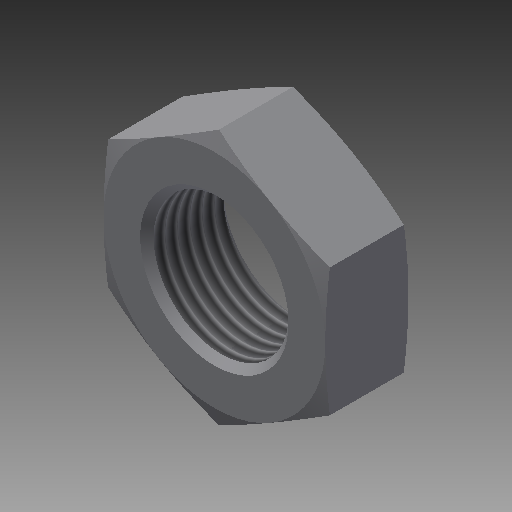
# Autodesk Inventor part: D-3556
Saved by Autodesk Inventor 2019 (Build 230136000, 136)
## iProperties
Category: PARTsolutions
Company: BIMBA
Created: 2019-01-13
Part Number: D-3556
Material: Generic
Catalog Web Link: www.cadenas.de
Description: Mounting Nut for Original Line Cylinders-
Vendor: BIMBA
Document SubType Name: Modeling
Designer: psadmin
Manufacturer: BIMBA
Mass: 4.89558 g
Surface Area: 24.7389 cm^2
Volume: 4.89558 cm^3
Density: 1 g/cm^3
Appearance: PSOLRGB-191-191-191
PSOL_IDENT_0: {$CADENAS_DATA\23d-libs\bimba\bimba\bimba_imperial\bimba_full_line\original_line_cylinders\accessori
PSOL_IDENT_1: es\mounting_nut.prj},189 {VTYP=3D},{NB=D-3556},{LINA=D-3556},{NN=Mounting Nut for Original Line Cyli
PSOL_IDENT_2: nders},{DATE=27.12.2018 09:32:42},{GEOMDATE=10.11.2011 00:00:00},{VERSION=},{LINEID=70},{WBVAR=MAT},
PSOL_IDENT_3: {WBNUMERIC=}  {NB=D-3556},{LINA=D-3556},{KT=DUMMY},{PN=D-3556},{PN1=D-3556},{C=3/4-16},{TH=UNF},{MAT=
PSOL_IDENT_4: },{MAT1='','Zinc-Plated Carbon Steel', '-SS', 'Stainless Steel'},{A=1.12},{A1=1.12000000},{B=0.42},{
PSOL_IDENT_5: B1=0.42000000},{NDM=0.75000000},{PITCH=0.0625},{DIA=-},{DIA2=-},{DIA3=-},{DIA1=0},{DIA4=0.00000000},
PSOL_IDENT_6: {DIA5=0.00000000},{T=-},{T2=-},{T3=-},{T1=0},{T4=0.00000000},{T5=0.00000000},{COLOR=0.75,0.75,0.75,0
PSOL_IDENT_7: .00},{TT=0.05000000},{TO=0.25000000},{PRA=1}
NN: Mounting Nut for Original Line Cylinders
NB: D-3556
NBSYN: $PN.
LINA: D-3556
PN: D-3556
C: 3/4-16
MAT: Zinc-Plated Carbon Steel
A: 1.12
B: 0.42
DIA: -
T: -
SUPPLIER: BIMBA
ARTICLENO: D-3556
BOMINFO: D-3556
CREATOR: CADENAS GmbH
Title: D-3556
Author: Cadenas PARTsolutions
Autodesk Inventor part; units mm, degrees
sketch "Sketch_8" plane through (0, 0, 0) normal (1, 0, 0) x (0, 1, 0)
  line L0 (0, -10.668) -> (0, 0)
  line L1 (0, 0) -> (14.224, 0)
  line L2 (14.224, 0) -> (17.0688, -0.7623)
  line L3 (17.0688, -0.7623) -> (17.0688, -9.9057)
  line L4 (17.0688, -9.9057) -> (14.224, -10.668)
  line L5 (14.224, -10.668) -> (0, -10.668)
  line L6 (0, -10.668) -> (0, 0)
  constraints: 14 end point
sketch "Sketch_10" plane through (0, 0, 0) normal (0, 0, 1) x (1, 0, 0)
  line L0 (-28.448, -28.448) -> (28.448, -28.448)
  line L1 (28.448, -28.448) -> (28.448, 28.448)
  line L2 (28.448, 28.448) -> (-28.448, 28.448)
  line L3 (-28.448, 28.448) -> (-28.448, -28.448)
  line L4 (-14.224, -8.2122) -> (0, -16.4245)
  line L5 (0, -16.4245) -> (14.224, -8.2122)
  line L6 (14.224, -8.2122) -> (14.224, 8.2122)
  line L7 (14.224, 8.2122) -> (0, 16.4245)
  line L8 (0, 16.4245) -> (-14.224, 8.2122)
  line L9 (-14.224, 8.2122) -> (-14.224, -8.2122)
  constraints: 20 end point
revolve "Revolution1" add sketch "Sketch_8" angle 360 about axis through (0, 0, -10.668) along (0, 0, -1)
extrude "Extrusion1" cut sketch "Sketch_10" against normal blind 10.668
sketch "Sketch_11" plane through (0, 0, 0) normal (1, 0, 0) x (0, 1, 0)
  line L0 (0, -10.668) -> (0, 0)
  line L1 (0, 0) -> (9.525, 0)
  line L2 (9.525, 0) -> (8.6652, -0.8598)
  line L3 (8.6652, -0.8598) -> (8.6652, -9.8082)
  line L4 (8.6652, -9.8082) -> (9.525, -10.668)
  line L5 (9.525, -10.668) -> (0, -10.668)
  line L6 (0, -10.668) -> (0, 0)
  constraints: 14 end point
revolve "Revolution2" cut sketch "Sketch_11" angle 360 about axis through (0, 0, -10.668) along (0, 0, -1)
thread "Thread1" size "3/4-16 UNF" class "2B" standard "ANSI Unified Screw Threads" full length
ref_plane "NUT_XY" through (0, 0, 0) normal (0, 0, 1) x (1, 0, 0)
ref_plane "NUT_YZ" through (0, 0, 0) normal (1, 0, 0) x (0, 1, 0)
ref_plane "NUT_ZX" through (0, 0, 0) normal (0, 1, 0) x (0, 0, 1)
ref_plane "a1_XY" through (-14.224, 14.224, 0) normal (0, 0, 1) x (1, 0, 0)
ref_plane "a1_YZ" through (-14.224, 14.224, 0) normal (1, 0, 0) x (0, 1, 0)
ref_plane "a1_ZX" through (-14.224, 14.224, 0) normal (0, 1, 0) x (0, 0, 1)
ref_plane "a2_XY" through (14.224, 14.224, 0) normal (0, 0, 1) x (1, 0, 0)
ref_plane "a2_YZ" through (14.224, 14.224, 0) normal (1, 0, 0) x (0, 1, 0)
ref_plane "a2_ZX" through (14.224, 14.224, 0) normal (0, 1, 0) x (0, 0, 1)
ref_plane "b1_XY" through (0, 14.224, 0) normal (1, 0, 0) x (0, 0, -1)
ref_plane "b1_YZ" through (0, 14.224, 0) normal (0, 0, -1) x (0, 1, 0)
ref_plane "b1_ZX" through (0, 14.224, 0) normal (0, 1, 0) x (1, 0, 0)
ref_plane "b2_XY" through (0, 14.224, -10.668) normal (1, 0, 0) x (0, 0, -1)
ref_plane "b2_YZ" through (0, 14.224, -10.668) normal (0, 0, -1) x (0, 1, 0)
ref_plane "b2_ZX" through (0, 14.224, -10.668) normal (0, 1, 0) x (1, 0, 0)
ref_plane "e_XY" through (0, 0, -10.668) normal (1, 0, 0) x (0, 0, -1)
ref_plane "e_YZ" through (0, 0, -10.668) normal (0, 0, -1) x (0, 1, 0)
ref_plane "e_ZX" through (0, 0, -10.668) normal (0, 1, 0) x (1, 0, 0)
ref_plane "ol1_XY" through (0, 0, -14.224) normal (0, 1, 0) x (1, 0, 0)
ref_plane "ol1_YZ" through (0, 0, -14.224) normal (1, 0, 0) x (0, 0, -1)
ref_plane "ol1_ZX" through (0, 0, -14.224) normal (0, 0, -1) x (0, 1, 0)
ref_plane "ol2_XY" through (10.668, 0, -14.224) normal (0, 1, 0) x (1, 0, 0)
ref_plane "ol2_YZ" through (10.668, 0, -14.224) normal (1, 0, 0) x (0, 0, -1)
ref_plane "ol2_ZX" through (10.668, 0, -14.224) normal (0, 0, -1) x (0, 1, 0)
ref_plane "th1_XY" through (0, 9.525, -10.668) normal (1, 0, 0) x (0, 0, -1)
ref_plane "th1_YZ" through (0, 9.525, -10.668) normal (0, 0, -1) x (0, 1, 0)
ref_plane "th1_ZX" through (0, 9.525, -10.668) normal (0, 1, 0) x (1, 0, 0)
ref_plane "th2_XY" through (0, -9.525, -10.668) normal (1, 0, 0) x (0, 0, -1)
ref_plane "th2_YZ" through (0, -9.525, -10.668) normal (0, 0, -1) x (0, 1, 0)
ref_plane "th2_ZX" through (0, -9.525, -10.668) normal (0, 1, 0) x (1, 0, 0)
body "Solid1"
